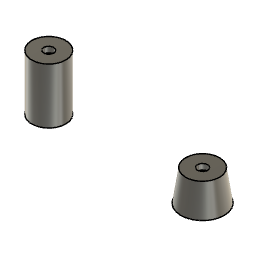
ThreadedRodConnectors v12 (Autodesk Fusion 360 design; units mm, degrees)
Autodesk Fusion 360 part; units mm, degrees
sketch "BaseSketch" plane through (0, 0, 0) normal (0, 0, 1) x (1, 0, 0)
  circle A0 centre (0, 0) radius 5.5
  circle A1 centre (0, 0) radius 1.6
  dimension "d63" = 11
  dimension "d64" = 3.2
  constraint coincident A0.centre A1.centre
  constraint concentric A0 A1
  measures "d63" diameter of A0
  measures "d64" diameter of A1
extrude "ExtrudeCylinder" add sketch "BaseSketch" along normal blind 18 makes body 1
sketch "Nut4mmSketch" plane through (0, 0, 0) normal (0, 0, -1) x (1, 0, 0)
  circle A0 centre (0, 0) radius 1.6
  circle A1 centre (0, 0) radius 5.5
  line L0 (2.85, 1.6454) -> (0, 3.2909)
  line L1 (0, 3.2909) -> (-2.85, 1.6454)
  line L2 (-2.85, 1.6454) -> (-2.85, -1.6454)
  line L3 (-2.85, -1.6454) -> (0, -3.2909)
  line L4 (0, -3.2909) -> (2.85, -1.6454)
  line L5 (2.85, -1.6454) -> (2.85, 1.6454)
  dimension "d68" = 2.85
  constraint coincident A0.centre A1.centre
  constraint vertical L5
  measures "d68" distance of A0.centre L5
sketch "Nut3mmSketch" plane through (0, 0, 18) normal (0, 0, 1) x (-1, 0, 0)
  circle A0 centre (0, 0) radius 1.6
  circle A1 centre (0, 0) radius 5.5
  line L0 (2.85, 1.6454) -> (0, 3.2909)
  line L1 (0, 3.2909) -> (-2.85, 1.6454)
  line L2 (-2.85, 1.6454) -> (-2.85, -1.6454)
  line L3 (-2.85, -1.6454) -> (0, -3.2909)
  line L4 (0, -3.2909) -> (2.85, -1.6454)
  line L5 (2.85, -1.6454) -> (2.85, 1.6454)
  dimension "d69" = 2.85
  constraint coincident A0.centre A1.centre
  constraint vertical L5
  measures "d69" distance of A0.centre L5
extrude "Cut4mmNut" cut sketch "Nut4mmSketch" against normal blind 2.2 from surface at -1.2 contours L0 L1 L2 L3 L4 L5 bodies 1
extrude "Cut3mmNut" cut sketch "Nut3mmSketch" against normal blind 2.2 from surface at -3 contours L0 L1 L2 L3 L4 L5 bodies 1
sketch "BigHoleSketch" plane through (0, 0, 0) normal (0, 0, -1) x (1, 0, 0)
  circle A0 centre (0, 0) radius 1.6
  circle A1 centre (0, 0) radius 5.5
  circle A2 centre (0, 0) radius 5.5
  circle A3 centre (0, 0) radius 2.1
  dimension "d77" = 11
  dimension "d78" = 4.2
  constraint coincident A0.centre A1.centre
  constraint concentric A0 A3
  measures "d77" diameter of A2
  measures "d78" diameter of A3
sketch "Taper4mm" plane through (0, 0, 3.4) normal (0, 0, -1) x (1, 0, 0)
  circle A0 centre (0, 0) radius 1.6
  line L0 (2.85, -1.6454) -> (2.85, 1.6454)
  line L1 (2.85, 1.6454) -> (0, 3.2909)
  line L2 (0, 3.2909) -> (-2.85, 1.6454)
  line L3 (-2.85, 1.6454) -> (-2.85, -1.6454)
  line L4 (-2.85, -1.6454) -> (0, -3.2909)
  line L5 (0, -3.2909) -> (2.85, -1.6454)
  circle A1 centre (0, 0) radius 2.75
  dimension "d85" = 5.5
  constraint coincident A0.centre A1.centre
  measures "d85" diameter of A1
extrude "CutTaper4mm" cut sketch "Taper4mm" against normal blind 10 draft -40 contours A0 | A1 bodies 1
sketch "Taper3mm" plane through (0, 0, 15) normal (0, 0, -1) x (1, 0, 0)
  circle A0 centre (0, 0) radius 1.6
  line L0 (-2.85, 1.6454) -> (-2.85, -1.6454)
  line L1 (-2.85, -1.6454) -> (0, -3.2909)
  line L2 (0, -3.2909) -> (2.85, -1.6454)
  line L3 (2.85, -1.6454) -> (2.85, 1.6454)
  line L4 (2.85, 1.6454) -> (0, 3.2909)
  line L5 (0, 3.2909) -> (-2.85, 1.6454)
  circle A1 centre (0, 0) radius 2.75
  dimension "d88" = 5.5
  constraint coincident A0.centre A1.centre
  measures "d88" diameter of A1
extrude "CutTaper3mm" cut sketch "Taper3mm" against normal blind 3 draft -45 contours A0 | A1 bodies 1
sketch "BottomSketch" plane through (0, 0, 0) normal (0, 0, 1) x (1, 0, 0) in component "Striker"
  circle A0 centre (50, 0) radius 7
  point P0 (50, 0)
  dimension "d93" = 14
  dimension "d96" = 50
  constraint coincident P0 A0.centre
  constraint horizontal origin A0.centre
  measures "d93" diameter of A0
  measures "d96" distance of origin A0.centre
ref_plane "WorkPlane1" through (50, 0, 10) normal (0, 0, 1) x (1, 0, 0) in component "Striker"
sketch "TopSketch" plane through (0, 0, 10) normal (0, 0, 1) x (1, 0, 0) in component "Striker"
  circle A0 centre (50, 0) radius 5.5
  circle A1 centre (50, 0) radius 1.6
  point P0 (50, 0)
  dimension "d95" = 11
  dimension "d97" = 3.2
  constraint coincident P0 A0.centre
  constraint concentric A0 A1
  measures "d95" diameter of A0
  measures "d97" diameter of A1
loft "LoftBody" add profiles "BottomSketch", "TopSketch" section 1 section 2 contours A0 | A1 separate body makes body 2 in component "Striker"
extrude "Extrude1" cut sketch "TopSketch" against normal up to surface (8 mm away) contours A1 bodies 2 in component "Striker"
sketch "NutSketch" plane through (0, 0, 10) normal (0, 0, 1) x (1, 0, 0) in component "Striker"
  line L0 (47.15, -1.6454) -> (50, -3.2909)
  line L1 (50, -3.2909) -> (52.85, -1.6454)
  line L2 (52.85, -1.6454) -> (52.85, 1.6454)
  line L3 (52.85, 1.6454) -> (50, 3.2909)
  line L4 (50, 3.2909) -> (47.15, 1.6454)
  line L5 (47.15, 1.6454) -> (47.15, -1.6454)
  point P0 (50, 0)
  point P1 (50, 0)
  dimension "d100" = 2.85
  constraint coincident P1 P0
  constraint vertical L2
  measures "d100" distance of P1 L5
extrude "CutNutHole" cut sketch "NutSketch" against normal blind 2.2 from surface at -3 bodies 2 in component "Striker"
sketch "NutCone" plane through (0, 0, 7) normal (0, 0, -1) x (1, 0, 0) in component "Striker"
  circle A0 centre (50, 0) radius 1.6
  line L0 (47.15, 1.6454) -> (47.15, -1.6454)
  line L1 (47.15, -1.6454) -> (50, -3.2909)
  line L2 (50, -3.2909) -> (52.85, -1.6454)
  line L3 (52.85, -1.6454) -> (52.85, 1.6454)
  line L4 (52.85, 1.6454) -> (50, 3.2909)
  line L5 (50, 3.2909) -> (47.15, 1.6454)
  circle A1 centre (50, 0) radius 2.75
  dimension "d104" = 5.5
  constraint concentric A0 A1
  measures "d104" diameter of A1
extrude "Extrude3" cut sketch "NutCone" against normal blind 4 draft -45 contours A0 | A1 bodies 2 in component "Striker"
component "Striker" placed x (1, 0, 0) y (0, 1, 0) z (0, 0, 1) at (0, 0, 0)
equation "nut_thickness = 2.6 mm"
equation "outer_diam = 11 mm"
equation "inner_diam_small = 3.2 mm"
equation "nut3mm_circumscribe = 2.85 mm"
equation "nut4mm_circumscribe = 3.6 mm"
equation "nut3mm_thickness = 2.2 mm"
equation "nut4mm_thickness = 3.2 mm"
equation "nut3mm_dist = 3 mm"
equation "nut4mm_dist = 1.2 mm"
equation "d63 = outer_diam"
equation "d64 = inner_diam_small"
equation "total_height = 18 mm"
equation "d66 = total_height"
equation "d68 = nut3mm_circumscribe"
equation "d69 = nut3mm_circumscribe"
equation "d70 = -nut4mm_dist"
equation "d71 = -nut3mm_thickness"
equation "d73 = -nut3mm_dist"
equation "d74 = -nut3mm_thickness"
equation "inner_diam_large = 4.2 mm"
equation "d77 = outer_diam"
equation "d78 = inner_diam_large"
equation "d85 = nut3mm_circumscribe * 2 - 0.2 mm"
equation "d88 = nut3mm_circumscribe * 2 - 0.2 mm"
equation "striker_base_diam = 14 mm"
equation "striker_height = 10 mm"
equation "d93 = striker_base_diam"
equation "d94 = striker_height"
equation "d95 = outer_diam"
equation "d97 = inner_diam_small"
equation "d100 = nut3mm_circumscribe"
equation "d101 = -nut3mm_dist"
equation "d102 = -nut3mm_thickness"
equation "d104 = ( nut3mm_circumscribe * 2 ) - 0.2 mm"
named bodies: "SolenoidToRodAttachment", "Striker"
